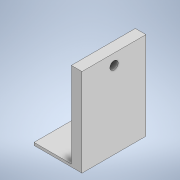
# Autodesk Inventor part: oneHalfForkSupport
Saved by Autodesk Inventor 2021 (Build 250183000, 183)
## iProperties
Created: 2020-06-25
Part Number: oneHalfForkSupport
Material: Generic
Document SubType Name: Modeling
Designer: robst
Density: 1 g/cm^3
Appearance: Default
Author: robst
Autodesk Inventor part; units mm, degrees
ref_plane "YZ Plane" through (0, 0, 0) normal (1, 0, 0) x (0, 1, 0)
ref_plane "XZ Plane" through (0, 0, 0) normal (0, 1, 0) x (-1, 0, 0)
ref_plane "XY Plane" through (0, 0, 0) normal (0, 0, 1) x (1, 0, 0)
sketch "Sketch2" plane through (0, 0, 0) normal (0, 1, 0) x (-1, 0, 0)
  line L0 (0, 0) -> (-114.3, 0)
  line L1 (-114.3, 0) -> (-114.3, -152.4)
  line L2 (-114.3, -152.4) -> (0, -152.4)
  line L3 (0, -152.4) -> (0, 0)
  dimension "d1" = 152.4
  dimension "d2" = 114.3
  constraints: 8 end point, 2 parallel, 1 horizontal, 1 perpendicular
  measures "d1" distance of L2.end L0.start
  measures "d2" distance of L1.end L2.end
extrude "Extrusion1" add sketch "Sketch2" against normal blind 6.35
sketch "Sketch3" plane through (0, 0, 0) normal (0, 1, 0) x (1, 0, 0)
  line L0 (114.3, 0) -> (114.3, 152.4) projected
  line L1 (114.3, 152.4) -> (0, 152.4) projected
  line L2 (0, 0) -> (114.3, 0) projected
  line L3 (114.3, 152.4) -> (114.3, 0) projected
  line L4 (0, 152.4) -> (114.3, 152.4) projected
  line L5 (114.3, 0) -> (88.9, 0)
  line L6 (88.9, 0) -> (88.9, 152.4)
  line L7 (88.9, 152.4) -> (114.3, 152.4)
  line L8 (114.3, 152.4) -> (114.3, 0)
  point P0 (88.9, 0)
  dimension "d5" = 25.4
  constraints: 8 end point, 2 parallel, 1 horizontal, 1 perpendicular, 1 point on line
  measures "d5" distance between parallel lines of L6 L0
extrude "Extrusion2" add sketch "Sketch3" along normal blind 203.2
sketch "Sketch4" plane through (114.3, -6.35, 0) normal (1, 0, 0) x (0, 0, -1)
  line L0 (0, 209.55) -> (152.4, 209.55) construction
  line L1 (76.2, 209.55) -> (76.2, 0) construction
  line L2 (152.4, 0) -> (0, 0) construction
  point P0 (0, 6.35)
  point P1 (76.2, 184.15)
  dimension "d8" = 25.4
  constraints: 2 end point, 2 midpoint, 1 point on line
  measures "d8" distance from line of point (76.2, 184.15) L0
hole "Hole1" at (114.3, 177.8, -76.2) direction (-1, 0, 0) diameter 19.8374 end through all
body "Solid1"
